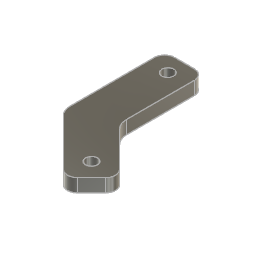
handle v4 (Autodesk Fusion 360 design; units mm, degrees)
Autodesk Fusion 360 part; units mm, degrees
sketch "Sketch1" plane through (0, 0, 0) normal (0, 0, 1) x (1, 0, 0)
  line L0 (0, -3) -> (0, -28.4142)
  line L1 (3, 0) -> (9, 0)
  line L2 (12, -3) -> (12, -23.4437)
  circle A0 centre (6, -5) radius 1.8
  arc A1 (3, 0) -> (0, -3) centre (3, -3) ccw
  arc A2 (12, -3) -> (9, 0) centre (9, -3) ccw
  line L3 (13.4645, -26.9792) -> (24.0208, -37.5355)
  line L4 (24.0208, -41.7782) -> (19.7782, -46.0208)
  line L5 (15.5355, -46.0208) -> (1.4645, -31.9497)
  arc A3 (24.0208, -41.7782) -> (24.0208, -37.5355) centre (21.8995, -39.6569) ccw
  arc A4 (15.5355, -46.0208) -> (19.7782, -46.0208) centre (17.6569, -43.8995) ccw
  arc A5 (12, -23.4437) -> (13.4645, -26.9792) centre (17, -23.4437) ccw
  arc A6 (0, -28.4142) -> (1.4645, -31.9497) centre (5, -28.4142) ccw
  circle A7 centre (17.6569, -39.6569) radius 1.8
  point P0 (0, -25)
  point P1 (12, 0)
  point P2 (12, -25)
  point P3 (12, -25.5147)
  point P4 (26.1421, -39.6569)
  point P5 (17.6569, -48.1421)
  dimension "d19" = 25
  dimension "d22" = 12
  dimension "d23" = 25
  dimension "d25" = 3.6
  dimension "d26" = 6
  dimension "d27" = 5
  dimension "d30" = 3
  dimension "d31" = 3
  dimension "d41" = 20
  dimension "d42" = 135
  dimension "d43" = 12
  dimension "d44" = 135
  dimension "d45" = 3
  dimension "d46" = 5
  dimension "d47" = 5
  dimension "d48" = 3.6
  dimension "d49" = 6
  dimension "d50" = 6
  constraint vertical L0
  constraint perpendicular L0 L1
  constraint perpendicular L1 L2
  constraint coincident origin L1
  constraint coincident origin L0
  constraint tangent L1 A1
  constraint tangent L0 A1
  constraint coincident P1 L1
  constraint coincident P1 L2
  constraint tangent L1 A2
  constraint tangent L2 A2
  constraint coincident P0 L0
  constraint coincident P2 L2
  constraint perpendicular L3 L4
  constraint coincident P4 L3
  constraint coincident P4 L4
  constraint tangent L3 A3
  constraint tangent L4 A3
  constraint coincident P5 L4
  constraint coincident P5 L5
  constraint tangent L4 A4
  constraint tangent L5 A4
  constraint equal A3 A4
  constraint coincident L2 P3
  constraint coincident P3 L3
  constraint tangent L2 A5
  constraint tangent L3 A5
  constraint tangent L0 A6
  constraint tangent L5 A6
  measures "d19" distance of origin P0
  measures "d22" distance of origin P1
  measures "d23" distance of P1 P2
  measures "d25" diameter of A0
  measures "d26" distance of L0 A0.centre
  measures "d27" distance of L1 A0.centre
  measures "d30" radius of A1
  measures "d31" radius of A2
  measures "d41" distance of P3 P4
  measures "d42" angle of L2 L3
  measures "d43" distance of P4 P5
  measures "d44" angle of L0 L5
  measures "d45" radius of A3
  measures "d46" radius of A5
  measures "d47" radius of A6
  measures "d48" diameter of A7
  measures "d49" distance of L4 A7.centre
  measures "d50" distance of L3 A7.centre
extrude "Extrude2" add sketch "Sketch1" along normal blind 4
